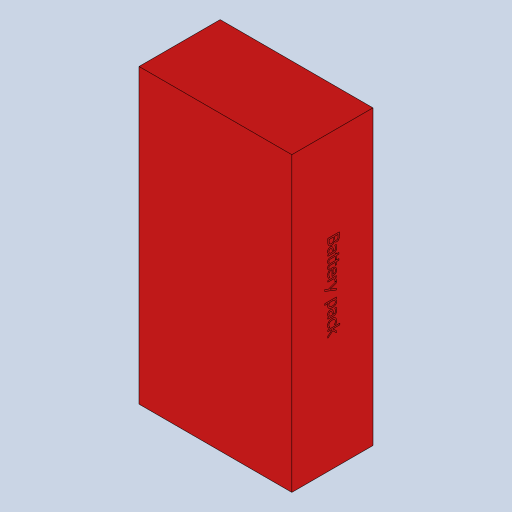
# Autodesk Inventor part: Battery pack
Saved by Autodesk Inventor 2024 (Build 280153000, 153)
## iProperties
Created: 2024-04-23
Part Number: Battery pack
Material: Generic
Document SubType Name: Modeling
Designer: mirun
Density: 1 g/cm^3
Appearance: Default
Author: mirun
Autodesk Inventor part; units mm, degrees
ref_plane "YZ Plane" through (0, 0, 0) normal (1, 0, 0) x (0, 1, 0)
ref_plane "XZ Plane" through (0, 0, 0) normal (0, 1, 0) x (-1, 0, 0)
ref_plane "XY Plane" through (0, 0, 0) normal (0, 0, 1) x (1, 0, 0)
sketch "Sketch1" plane through (0, 0, 0) normal (0, 1, 0) x (-1, 0, 0)
  line L0 (-20.25, 10.75) -> (20.25, 10.75)
  line L1 (20.25, 10.75) -> (20.25, -10.75)
  line L2 (20.25, -10.75) -> (-20.25, -10.75)
  line L3 (-20.25, -10.75) -> (-20.25, 10.75)
  line L4 (-20.25, 10.75) -> (20.25, -10.75) construction
  line L5 (20.25, 10.75) -> (-20.25, -10.75) construction
  point P0 (0, 0)
  point P1 (0, -10.75)
  dimension "d0" = 40.5
  dimension "d1" = 21.5
  constraints: 12 end point, 3 midpoint, 2 parallel, 1 horizontal, 1 perpendicular
  measures "d0" distance of L1.end L2.end
  measures "d1" distance from line of point (0, -10.75) L0
extrude "Extrusion1" add sketch "Sketch1" along normal blind 77.5
sketch "Sketch2" plane through (20.25, 0, 10.75) normal (1, 0, 0) x (0, 0, -1)
  line L0 (12.7144, 53.8105) -> (12.7144, 26.87) construction
  line L1 (12.7144, 26.87) -> (3.5472, 26.87) construction
  line L2 (3.5472, 26.87) -> (3.5472, 53.8105) construction
  line L3 (3.5472, 53.8105) -> (12.7144, 53.8105) construction
  point P0 (10.75, 0)
  constraints: 2 other
mark "Mark1"
body "Solid1"
